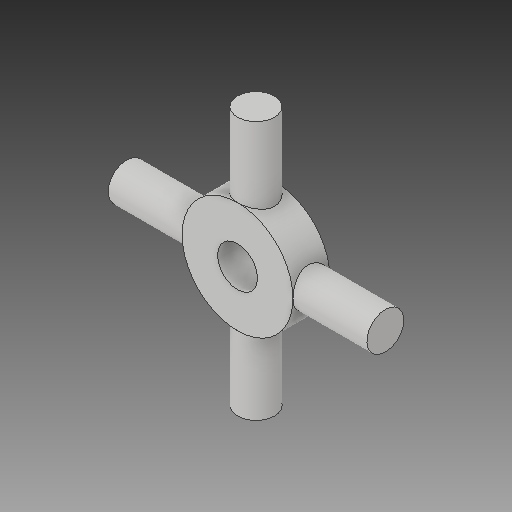
# Autodesk Inventor part: SweeperHub
Saved by Autodesk Inventor 2019 (Build 230136000, 136)
## iProperties
Created: 2018-12-01
Part Number: SweeperHub
Material: Generic
Document SubType Name: Modeling
Designer: User
Density: 1 g/cm^3
Appearance: Default
Author: User
Autodesk Inventor part; units mm, degrees
ref_plane "YZ Plane" through (0, 0, 0) normal (1, 0, 0) x (0, 1, 0)
ref_plane "XZ Plane" through (0, 0, 0) normal (0, 1, 0) x (-1, 0, 0)
sketch "Sketch1" plane through (0, 0, 0) normal (0, 1, 0) x (-1, 0, 0)
  circle A0 centre (0, 0) radius 3.175
  dimension "d0" = 6.35
  constraints: 1 centre point, 1 coincident
  measures "d0" diameter of A0
extrude "Extrusion1" add sketch "Sketch1" along normal blind 22.225
pattern_circular "Circular Pattern1" count 4 over 360 about axis through (0, 0, -10) along (0, 0, 1) of "Extrusion1"
sketch "Sketch2" plane through (0, 0, 0) normal (0, 0, 1) x (1, 0, 0)
  line L0 (0, 0) -> (3.175, -3.175) projected
  circle A0 centre (0, 0) radius 9.525
  dimension "d6" = 19.05
  constraints: 1 centre point, 1 coincident
  measures "d6" diameter of A0
extrude "Extrusion2" add sketch "Sketch2" along normal mid plane 6.35
sketch "Sketch3" plane through (0, 0, -3.175) normal (0, 0, -1) x (-1, 0, 0)
  point P0 (0, 0)
  point P1 (0, 0)
  constraints: 1 coincident
hole "Hole1" at (0, 0, -3.175) direction (0, 0, 1) diameter 6.858 depth 25.4 tip angle 118
sketch "Sketch4" plane through (0, 0, -3.175) normal (0, 0, -1) x (-1, 0, 0)
  line L0 (-3.175, 8.9803) -> (-3.175, 22.225) projected
  line L1 (-22.225, 3.175) -> (-8.9803, 3.175) projected
  arc A0 (0, 9.525) -> (-9.525, 0) centre (0, 0) ccw projected
  line L2 (-10.2954, 3.175) -> (-3.175, 10.2954)
  point P0 (0, 0)
  dimension "d16" = 45
  constraints: 2 end point, 2 point on line, 1 tangent
  measures "d16" angle of L1 L2
ref_plane "Work Plane1" through (10.2954, 3.175, -3.175) normal (0.7071, 0.7071, 0) x (-0.7071, 0.7071, 0)
sketch "Sketch5" plane through (10.2954, 3.175, -3.175) normal (0.7071, 0.7071, 0) x (-0.7071, 0.7071, 0)
  point P0 (5.0349, 3.175)
  point P1 (5.0349, 3.175)
  constraints: 1 coincident
body "Solid1"
